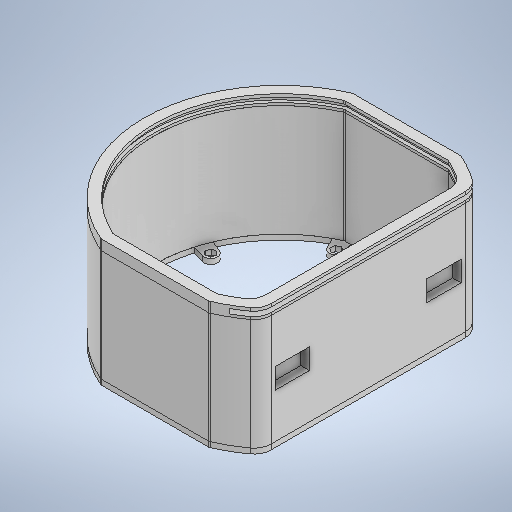
# Autodesk Inventor part: carcasa4.0
Saved by Autodesk Inventor 2025.3 (Build 293356030, 356C)
## iProperties
Created: 2025-08-27
Part Number: carcasa4.0
Material: Generic
Document SubType Name: Modeling
Designer: cdavi
Density: 1 g/cm^3
Appearance: Default
Author: cdavi
Autodesk Inventor part; units mm, degrees
ref_plane "YZ Plane" through (0, 0, 0) normal (1, 0, 0) x (0, 1, 0)
ref_plane "XZ Plane" through (0, 0, 0) normal (0, 1, 0) x (-1, 0, 0)
ref_plane "XY Plane" through (0, 0, 0) normal (0, 0, 1) x (1, 0, 0)
sketch "Sketch1" plane through (0, 0, 0) normal (0, 1, 0) x (-1, 0, 0)
  line L0 (29.8957, 67.5) -> (-29.8957, 67.5)
  line L1 (0, 0) -> (-51, 0) construction
  line L2 (31.1729, 73.5) -> (-31.1729, 73.5)
  line L3 (29.8957, -67.5) -> (-30.3274, -67.5)
  line L4 (31.1729, -73.5) -> (-31.1729, -73.5)
  line L5 (0, 0) -> (0, 73.5) construction
  line L6 (-45, 53.5817) -> (-45, -53.5817)
  line L7 (-51, 56.7362) -> (-51, -56.7362)
  arc A0 (-40.4687, -61.9539) -> (-30.3274, -67.5) centre (0, 0) ccw
  arc A1 (-46.8571, -64.8414) -> (-31.9722, -73.3333) centre (0, 0) ccw
  arc A2 (31.9722, -73.3333) -> (31.9722, 73.3333) centre (0, 0) ccw
  arc A3 (-31.9722, 73.3333) -> (-46.8571, 64.8414) centre (0, 0) ccw
  arc A4 (30.7261, -67.3194) -> (30.7261, 67.3194) centre (0, 0) ccw
  arc A5 (-30.7261, 67.3194) -> (-40.4688, 61.9539) centre (0, 0) ccw
  arc A6 (-31.9722, -73.3333) -> (-31.1729, -73.5) centre (-31.1729, -71.5) ccw
  arc A7 (31.1729, -73.5) -> (31.9722, -73.3333) centre (31.1729, -71.5) ccw
  arc A8 (29.8957, -67.5) -> (30.7261, -67.3194) centre (29.8957, -65.5) ccw
  arc A9 (30.7261, 67.3194) -> (29.8957, 67.5) centre (29.8957, 65.5) ccw
  arc A10 (31.9722, 73.3333) -> (31.1729, 73.5) centre (31.1729, 71.5) ccw
  arc A11 (-29.8957, 67.5) -> (-30.7261, 67.3194) centre (-29.8957, 65.5) ccw
  arc A12 (-31.1729, 73.5) -> (-31.9722, 73.3333) centre (-31.1729, 71.5) ccw
  arc A13 (-40.4688, 61.9539) -> (-45, 53.5817) centre (-35, 53.5817) ccw
  arc A14 (-46.8571, 64.8414) -> (-51, 56.7362) centre (-41, 56.7362) ccw
  arc A15 (-51, -56.7362) -> (-46.8571, -64.8414) centre (-41, -56.7362) ccw
  arc A16 (-45, -53.5817) -> (-40.4687, -61.9539) centre (-35, -53.5817) ccw
  point P0 (-31.5872, 73.5)
  point P1 (30.3274, -67.5)
  point P2 (31.5872, -73.5)
  point P3 (-31.5872, -73.5)
  point P4 (-51, -61.636)
  point P5 (-45, 58.7452)
  point P6 (-45, -58.7452)
  point P7 (-51, 61.636)
  point P8 (31.5872, 73.5)
  point P9 (30.3274, 67.5)
  point P10 (-30.3274, 67.5)
  dimension "d2" = 67.5
  dimension "d4" = 6
  dimension "d6" = 45
  dimension "d7" = 6
  dimension "d8" = 2
  dimension "d9" = 10
  dimension "d10" = 74
  dimension "d11" = 80
  dimension "d12" = 74
  dimension "d13" = 80
  constraints: 45 point on circle, 22 tangent, 17 centre point, 16 end point, 11 point on line, 9 equal radius, 4 symmetric about line, 3 vertical, 2 coincident, 2 horizontal, 2 midpoint, 1 parallel
  measures "d2" distance between parallel lines of L1 L0
  measures "d4" distance between parallel lines of L0 L2
  measures "d6" distance between parallel lines of L6 L5
  measures "d7" distance between parallel lines of L7 L6
  measures "d8" radius of A6
  measures "d9" radius of A13
  measures "d10" radius of A4
  measures "d11" radius of A2
  measures "d12" radius of A0
  measures "d13" radius of A1
extrude "Extrusion1" add sketch "Sketch1" along normal blind 65
sketch "Sketch2" plane through (51, 0, 56.7362) normal (1, 0, 0) x (0, 0, -1)
  line L0 (56.7362, 0) -> (56.7362, 65) construction
  line L1 (110.3179, 65) -> (3.1545, 65) projected
  line L2 (2.4029, 38) -> (22.4029, 38)
  line L3 (22.4029, 38) -> (22.4029, 26)
  line L4 (22.4029, 26) -> (2.4029, 26)
  line L5 (2.4029, 26) -> (2.4029, 38)
  line L6 (0, 0) -> (113.4725, 0) projected
  line L7 (-16.5971, 0) -> (-16.5971, 65) projected
  line L8 (111.0696, 38) -> (91.0696, 38)
  line L9 (91.0696, 38) -> (91.0696, 26)
  line L10 (91.0696, 26) -> (111.0696, 26)
  line L11 (111.0696, 26) -> (111.0696, 38)
  dimension "d16" = 26
  dimension "d17" = 19
  dimension "d18" = 12
  dimension "d19" = 20
  constraints: 18 end point, 4 symmetric about line, 2 parallel, 1 horizontal, 1 midpoint, 1 perpendicular
  measures "d16" distance between parallel lines of L6 L4
  measures "d17" distance between parallel lines of L5 L7
  measures "d18" distance of L2.end L3.end
  measures "d19" distance of L2.start L2.end
extrude "Extrusion2" cut sketch "Sketch2" against normal blind 5
sketch "Sketch3" plane through (51, 0, 56.7362) normal (1, 0, 0) x (0, 0, -1)
  line L0 (3.568, 49.2223) -> (17.7975, 43.9952) construction
  line L1 (2.8909, 47.379) -> (17.1204, 42.1519)
  line L2 (18.4746, 45.8385) -> (4.2452, 51.0656)
  arc A0 (4.2452, 51.0656) -> (2.8909, 47.379) centre (3.568, 49.2223) ccw
  arc A1 (17.1204, 42.1519) -> (18.4746, 45.8385) centre (17.7975, 43.9952) ccw
  arc A2 (44.4296, 11.624) -> (34.6921, 2.9774) centre (43.8866, 2.4292) ccw construction
  arc A3 (44.531, 13.3402) -> (32.9759, 3.0797) centre (43.8866, 2.4292) ccw
  arc A4 (44.3283, 9.9077) -> (36.4083, 2.8751) centre (43.8866, 2.4292) ccw
  arc A5 (44.3283, 9.9077) -> (44.531, 13.3402) centre (44.4296, 11.624) ccw
  arc A6 (32.9759, 3.0797) -> (36.4083, 2.8751) centre (34.6921, 2.9774) ccw
  line L3 (56.7362, 0) -> (56.7362, 65) construction
  line L4 (110.5816, 47.379) -> (96.3521, 42.1519)
  line L5 (94.9978, 45.8385) -> (109.2273, 51.0656)
  arc A7 (110.5816, 47.379) -> (109.2273, 51.0656) centre (109.9044, 49.2223) ccw
  arc A8 (94.9978, 45.8385) -> (96.3521, 42.1519) centre (95.675, 43.9952) ccw
  point P0 (10.6828, 46.6088)
  constraints: 18 point on circle, 12 end point, 9 centre point, 8 tangent, 6 symmetric about line, 1 midpoint, 1 parallel, 2 other
extrude "Extrusion3" [suppressed]
extrude "Extrusion4" add sketch "Sketch1" along normal blind 3 from surface at 65 separate body contours A9 A4 A8 L3 A0 A16 L6 A13 A5 A11 L0 | A10 A2 A7 L4 A6 A1 A15 L7 A14 A3 A12 L2
sketch "Sketch5" plane through (-31.1729, 68, 73.5) normal (0, 1, 0) x (1, 0, 0)
  circle A0 centre (31.1729, 73.5) radius 8.5
  circle A1 centre (1.1729, 73.5) radius 2.5
  line L0 (39.2969, 71) -> (48.1729, 71)
  line L1 (48.1729, 71) -> (48.1729, 76)
  line L2 (48.1729, 76) -> (39.2969, 76)
  line L3 (48.1729, 73.5) -> (82.1729, 73.5)
  line L4 (82.1729, 16.7638) -> (82.1729, 130.2362) projected
  line L5 (1.1729, 73.5) -> (-48.8271, 73.5)
  arc A2 (-0.7993, 146.8333) -> (-0.7993, 0.1667) centre (31.1729, 73.5) ccw projected
  dimension "d26" = 17
  dimension "d27" = 5
  dimension "d31" = 5
  dimension "d32" = 17
  dimension "d47" = 30
  dimension "d204" = 34
  dimension "d205" = 50
  dimension "d206" = 51
  constraints: 10 end point, 3 point on circle, 2 centre point, 2 horizontal alignment, 2 midpoint, 2 perpendicular, 1 coincident, 1 horizontal, 1 point on line
  measures "d26" diameter of A0
  measures "d27" diameter of A1
  measures "d31" distance between parallel lines of L2 L0
  measures "d32" distance from line of A0.centre L1
  measures "d47" distance of A0.centre L5.start
  measures "d204" distance of L3.start L3.end
  measures "d205" distance of L5.start L5.end
  measures "d206" distance from line of L4 point (31.173, 73.5)
extrude "Extrusion5" cut sketch "Sketch5" against normal through all bodies 2
sketch "Sketch6" plane through (0, 0, 0) normal (0, 1, 0) x (-1, 0, 0)
  circle A0 centre (0, 0) radius 67 construction
  arc A1 (-30.7261, 67.3194) -> (-40.4688, 61.9539) centre (0, 0) ccw projected
  arc A2 (-40.4688, 61.9539) -> (-45, 53.5817) centre (-35, 53.5817) ccw projected
  line L0 (-45, -53.5817) -> (-45, 53.5817) projected
  arc A3 (-45, -53.5817) -> (-40.4687, -61.9539) centre (-35, -53.5817) ccw projected
  arc A4 (-40.4687, -61.9539) -> (-30.3274, -67.5) centre (0, 0) ccw projected
  line L1 (29.8957, -67.5) -> (-30.3274, -67.5) construction
  arc A5 (30.7261, -67.3194) -> (30.7261, 67.3194) centre (0, 0) ccw projected
  line L2 (-29.8957, 67.5) -> (29.8957, 67.5) construction
  line L3 (31.1729, 73.5) -> (-31.1729, 73.5) projected
  arc A6 (-31.9722, 73.3333) -> (-46.8571, 64.8414) centre (0, 0) ccw projected
  arc A7 (-46.8571, 64.8414) -> (-51, 56.7362) centre (-41, 56.7362) ccw projected
  line L4 (-51, 56.7362) -> (-51, -56.7362) projected
  arc A8 (-51, -56.7362) -> (-46.8571, -64.8414) centre (-41, -56.7362) ccw projected
  arc A9 (-46.8571, -64.8414) -> (-31.9722, -73.3333) centre (0, 0) ccw projected
  line L5 (-31.1729, -73.5) -> (31.1729, -73.5) projected
  arc A10 (31.9722, -73.3333) -> (31.9722, 73.3333) centre (0, 0) ccw projected
  arc A11 (-29.4268, 61.303) -> (-37.1875, 56.9306) centre (0, 0) ccw construction
  arc A12 (-37.1875, 56.9306) -> (-39, 53.5817) centre (-35, 53.5817) ccw construction
  line L6 (-39, 53.5817) -> (-39, -53.5817) construction
  arc A13 (-39, -53.5817) -> (-37.1875, -56.9306) centre (-35, -53.5817) ccw construction
  arc A14 (-37.1875, -56.9306) -> (-29.4268, -61.303) centre (0, 0) ccw construction
  line L7 (-28.5613, -61.5) -> (28.5613, -61.5) construction
  line L8 (-28.5613, 61.5) -> (28.5613, 61.5) construction
  arc A15 (29.4268, -61.303) -> (29.4268, 61.303) centre (0, 0) ccw construction
  arc A16 (-8.124, -2.5) -> (-8.124, 2.5) centre (0, 0) ccw projected
  line L9 (0, 0) -> (63.1919, 22.2662) construction
  line L10 (0, 0) -> (80, 0) construction
  circle A17 centre (63.1919, 22.2662) radius 2.85 construction
  line L11 (0, 0) -> (0, -67) construction
  circle A18 centre (28.3154, 60.7226) radius 2.85 construction
  line L12 (28.3154, 60.7226) -> (0, 0) construction
  circle A19 centre (-41.5, 20) radius 2.85 construction
  circle A20 centre (-28.3154, 60.7226) radius 2.85 construction
  line L13 (-28.3154, 60.7226) -> (0, 0) construction
  arc A21 (-28.5613, 61.5) -> (-29.4268, 61.303) centre (-28.5613, 59.5) ccw construction
  arc A22 (-29.4268, -61.303) -> (-28.5613, -61.5) centre (-28.5613, -59.5) ccw construction
  arc A23 (28.5613, -61.5) -> (29.4268, -61.303) centre (28.5613, -59.5) ccw construction
  arc A24 (29.4268, 61.303) -> (28.5613, 61.5) centre (28.5613, 59.5) ccw construction
  arc A25 (-31.9722, -73.3333) -> (-31.1729, -73.5) centre (-31.1729, -71.5) ccw projected
  arc A26 (31.1729, -73.5) -> (31.9722, -73.3333) centre (31.1729, -71.5) ccw projected
  arc A27 (31.9722, 73.3333) -> (31.1729, 73.5) centre (31.1729, 71.5) ccw projected
  arc A28 (-31.1729, 73.5) -> (-31.9722, 73.3333) centre (-31.1729, 71.5) ccw projected
  circle A29 centre (63.1919, -22.2662) radius 2.85 construction
  circle A30 centre (28.3154, -60.7226) radius 2.85 construction
  circle A31 centre (-41.5, -20) radius 2.85 construction
  circle A32 centre (-28.3154, -60.7226) radius 2.85 construction
  line L14 (30.7261, 60.6622) -> (30.7261, 67.3194)
  line L15 (-30.7261, 60.6622) -> (-30.7261, 67.3194)
  line L16 (30.7261, 67.3194) -> (-30.7261, 67.3194)
  line L17 (30.7261, -60.6622) -> (30.7261, -67.3194)
  line L18 (-30.7261, -60.6622) -> (-30.7261, -67.3194)
  line L19 (30.7261, -67.3194) -> (-30.7261, -67.3194)
  circle A33 centre (63.1919, 22.2662) radius 4
  circle A34 centre (28.3154, 60.7226) radius 4
  line L20 (60.3905, 22.7899) -> (62.2448, 24.9542)
  line L21 (62.2448, 24.9542) -> (65.0462, 24.4304)
  line L22 (65.0462, 24.4304) -> (65.9934, 21.7424)
  line L23 (65.9934, 21.7424) -> (64.1391, 19.5782)
  line L24 (64.1391, 19.5782) -> (61.3376, 20.1019)
  line L25 (61.3376, 20.1019) -> (60.3905, 22.7899)
  line L26 (25.9808, 59.0879) -> (25.7324, 61.9271)
  line L27 (25.7324, 61.9271) -> (28.067, 63.5618)
  line L28 (28.067, 63.5618) -> (30.65, 62.3573)
  line L29 (30.65, 62.3573) -> (30.8984, 59.5182)
  line L30 (30.8984, 59.5182) -> (28.5638, 57.8835)
  line L31 (28.5638, 57.8835) -> (25.9808, 59.0879)
  circle A35 centre (-41.5, 20) radius 4
  line L32 (-43.9682, 18.575) -> (-43.9682, 21.425)
  line L33 (-43.9682, 21.425) -> (-41.5, 22.85)
  line L34 (-41.5, 22.85) -> (-39.0318, 21.425)
  line L35 (-39.0318, 21.425) -> (-39.0318, 18.575)
  line L36 (-39.0318, 18.575) -> (-41.5, 17.15)
  line L37 (-41.5, 17.15) -> (-43.9682, 18.575)
  line L38 (-41.5, 24) -> (-45, 24)
  line L39 (-41.5, 16) -> (-45, 16)
  circle A36 centre (-28.3154, 60.7226) radius 4
  line L40 (-28.5638, 57.8835) -> (-30.8984, 59.5182)
  line L41 (-30.8984, 59.5182) -> (-30.65, 62.3573)
  line L42 (-30.65, 62.3573) -> (-28.067, 63.5618)
  line L43 (-28.067, 63.5618) -> (-25.7324, 61.9271)
  line L44 (-25.7324, 61.9271) -> (-25.9808, 59.0879)
  line L45 (-25.9808, 59.0879) -> (-28.5638, 57.8835)
  line L46 (-31.8886, 58.9247) -> (-35.0362, 65.1802)
  circle A37 centre (63.1919, -22.2662) radius 4
  circle A38 centre (28.3154, -60.7226) radius 4
  circle A39 centre (-41.5, -20) radius 4
  line L47 (-41.5, -24) -> (-45, -24)
  line L48 (-41.5, -16) -> (-45, -16)
  circle A40 centre (-28.3154, -60.7226) radius 4
  line L49 (-31.8886, -58.9247) -> (-35.0362, -65.1802)
  line L50 (60.3905, -22.7899) -> (62.2448, -24.9542)
  line L51 (62.2448, -24.9542) -> (65.0462, -24.4304)
  line L52 (65.0462, -24.4304) -> (65.9934, -21.7424)
  line L53 (65.9934, -21.7424) -> (64.1391, -19.5782)
  line L54 (64.1391, -19.5782) -> (61.3376, -20.1019)
  line L55 (61.3376, -20.1019) -> (60.3905, -22.7899)
  line L56 (25.9808, -59.0879) -> (25.7324, -61.9271)
  line L57 (25.7324, -61.9271) -> (28.067, -63.5618)
  line L58 (28.067, -63.5618) -> (30.65, -62.3573)
  line L59 (30.65, -62.3573) -> (30.8984, -59.5182)
  line L60 (30.8984, -59.5182) -> (28.5638, -57.8835)
  line L61 (28.5638, -57.8835) -> (25.9808, -59.0879)
  line L62 (-28.5638, -57.8835) -> (-30.8984, -59.5182)
  line L63 (-30.8984, -59.5182) -> (-30.65, -62.3573)
  line L64 (-30.65, -62.3573) -> (-28.067, -63.5618)
  line L65 (-28.067, -63.5618) -> (-25.7324, -61.9271)
  line L66 (-25.7324, -61.9271) -> (-25.9808, -59.0879)
  line L67 (-25.9808, -59.0879) -> (-28.5638, -57.8835)
  line L68 (-43.9682, -18.575) -> (-43.9682, -21.425)
  line L69 (-43.9682, -21.425) -> (-41.5, -22.85)
  line L70 (-41.5, -22.85) -> (-39.0318, -21.425)
  line L71 (-39.0318, -21.425) -> (-39.0318, -18.575)
  line L72 (-39.0318, -18.575) -> (-41.5, -17.15)
  line L73 (-41.5, -17.15) -> (-43.9682, -18.575)
  line L74 (61.7506, 25.9975) -> (68.283, 28.5208)
  line L75 (64.408, 18.4555) -> (71.0794, 20.5846)
  line L76 (31.8886, 58.9247) -> (35.0362, 65.1802)
  line L77 (61.7506, -25.9975) -> (68.283, -28.5208)
  line L78 (64.408, -18.4555) -> (71.0794, -20.5846)
  line L79 (31.8886, -58.9247) -> (35.0362, -65.1802)
  line L80 (-24.6413, 62.3041) -> (-27.4101, 68.7364)
  line L81 (24.6413, 62.3041) -> (27.4101, 68.7364)
  line L82 (-24.6413, -62.3041) -> (-27.4101, -68.7364)
  line L83 (24.6413, -62.3041) -> (27.4101, -68.7364)
  line L84 (-29.8957, 67.5) -> (-51, 67.5)
  line L85 (-51, 67.5) -> (-51, 56.7362)
  line L86 (-42.9389, 67.5) -> (-29.8957, 67.5)
  point P0 (-29.0129, -61.5)
  point P1 (30.7261, -60.6622)
  point P2 (-30.7261, -60.6622)
  point P3 (28.3154, 60.7226)
  point P4 (28.3154, 60.7226)
  point P5 (-30.7261, -67.3194)
  point P6 (-35.0362, -65.1802)
  point P7 (71.0794, -20.5846)
  point P8 (68.283, -28.5208)
  point P9 (35.0362, -65.1802)
  point P10 (-27.1107, 64.5369)
  point P11 (-27.1107, -64.5369)
  point P12 (27.1107, -64.5369)
  point P13 (27.1107, 64.5369)
  point P14 (-45, 21.9365)
  point P15 (-45, 18.0635)
  point P16 (-32.0117, 62.2515)
  point P17 (32.0117, -62.2515)
  point P18 (66.8707, -20.6956)
  point P19 (65.0736, -25.796)
  point P20 (-32.0117, -62.2515)
  point P21 (-45, -21.9365)
  point P22 (-45, -18.0635)
  point P23 (65.0736, 25.796)
  point P24 (66.8707, 20.6956)
  point P25 (32.0117, 62.2515)
  point P26 (25.828, -65.0609)
  point P27 (-25.828, -65.0609)
  point P28 (30.7261, -63.9146)
  point P29 (-26.8002, -67.3194)
  point P30 (26.8002, -67.3194)
  point P31 (26.8002, 67.3194)
  point P32 (-26.8002, 67.3194)
  point P33 (30.7261, 63.9146)
  point P34 (-30.7261, -63.9146)
  point P35 (-30.7261, 63.9146)
  dimension "d33" = 134
  dimension "d39" = 5.7
  dimension "d34" = 6
  dimension "d35" = 6
  dimension "d36" = 6
  dimension "d37" = 19.41
  dimension "d38" = 25
  dimension "d40" = 20
  dimension "d41" = 3.5
  dimension "d42" = 25
  dimension "d44" = 2
  dimension "d61" = 8
  dimension "d62" = 8
  dimension "d63" = 8
  dimension "d64" = 8
  dimension "d171" = 90
  dimension "d172" = 10.7638
  constraints: 162 end point, 52 symmetric about line, 38 point on circle, 20 centre point, 16 tangent, 10 coincident, 6 perpendicular, 4 point on line, 3 equal radius, 2 parallel, 2 vertical, 1 collinear, 1 horizontal, 93 other
  measures "d34" radial gap between concentric circles of A1 A11
  measures "d35" distance between parallel lines of L2 L8
  measures "d36" radial gap between concentric circles of A5 A15
  measures "d37" angle of L10 L9
  measures "d38" angle of L11 L12
  measures "d40" distance from line of point (-41.5, 20) L10
  measures "d41" distance from line of L0 point (-41.5, 20)
  measures "d42" angle of L11 L13
  measures "d44" radius of A21
  measures "d61" diameter of A33
  measures "d62" diameter of A34
  measures "d63" diameter of A35
  measures "d64" diameter of A36
  measures "d171" angle of L85 L84
  measures "d172" distance of L84.end L4.start
extrude "Extrusion6" add sketch "Sketch6" against normal blind 3 separate body contours L15 A36 L46 A1 | L16 L80 A36 L15 | A36 | L16 L14 A34 L81 | A5 L76 A34 L14 | A34 | L38 A35 L0 | A35 L0 | L0 A35 | A5 L75 A33 L74 | A35 L39 L0 | A33 | A5 L77 A37 L78 | L48 A39 L0 | A37 | A39 L0 | L0 A39 | A5 L17 A38 L79 | A39 L47 L0 | L19 L83 A38 L17 | A38 | L19 L18 A40 L82 | A4 L49 A40 L18 | A40 | A27 A10 A26 L5 A25 A9 A8 L4 A7 A6 A28 L3
sketch "Sketch14" plane through (0, 65, 0) normal (0, 1, 0) x (1, 0, 0)
  arc A0 (-31.9722, 73.3333) -> (-31.9722, -73.3333) centre (0, 0) ccw projected
  arc A1 (-31.9722, -73.3333) -> (-31.1729, -73.5) centre (-31.1729, -71.5) ccw projected
  line L0 (-31.1729, -73.5) -> (31.1729, -73.5) projected
  arc A2 (31.1729, -73.5) -> (31.9722, -73.3333) centre (31.1729, -71.5) ccw projected
  arc A3 (31.9722, -73.3333) -> (46.8571, -64.8414) centre (0, 0) ccw projected
  arc A4 (46.8571, -64.8414) -> (51, -56.7362) centre (41, -56.7362) ccw projected
  line L1 (51, -56.7362) -> (51, 56.7362) projected
  arc A5 (51, 56.7362) -> (46.8571, 64.8414) centre (41, 56.7362) ccw projected
  arc A6 (46.8571, 64.8414) -> (31.9722, 73.3333) centre (0, 0) ccw projected
  arc A7 (31.9722, 73.3333) -> (31.1729, 73.5) centre (31.1729, 71.5) ccw projected
  line L2 (31.1729, 73.5) -> (-31.1729, 73.5) projected
  arc A8 (-31.1729, 73.5) -> (-31.9722, 73.3333) centre (-31.1729, 71.5) ccw projected
  line L3 (-29.8957, 67.5) -> (30.3274, 67.5) projected
  arc A9 (40.4687, 61.9539) -> (30.3274, 67.5) centre (0, 0) ccw projected
  arc A10 (45, 53.5817) -> (40.4687, 61.9539) centre (35, 53.5817) ccw projected
  line L4 (45, 53.5817) -> (45, -53.5817) projected
  arc A11 (40.4688, -61.9539) -> (45, -53.5817) centre (35, -53.5817) ccw projected
  arc A12 (30.7261, -67.3194) -> (40.4688, -61.9539) centre (0, 0) ccw projected
  arc A13 (29.8957, -67.5) -> (30.7261, -67.3194) centre (29.8957, -65.5) ccw projected
  line L5 (29.8957, -67.5) -> (-29.8957, -67.5) projected
  arc A14 (-30.7261, -67.3194) -> (-29.8957, -67.5) centre (-29.8957, -65.5) ccw projected
  arc A15 (-30.7261, 67.3194) -> (-30.7261, -67.3194) centre (0, 0) ccw projected
  arc A16 (-29.8957, 67.5) -> (-30.7261, 67.3194) centre (-29.8957, 65.5) ccw projected
extrude "Extrusion11" add sketch "Sketch14" along normal blind 6 separate body
sketch "Sketch15" plane through (51, 65, 56.7362) normal (1, 0, 0) x (0, 0, -1)
  line L0 (56.7362, 6) -> (56.7362, 0)
  line L1 (56.7362, 6) -> (0, 6)
  line L2 (0, 6) -> (-12.763, 6)
  line L3 (-12.763, 6) -> (-12.763, 0)
  line L4 (-12.763, 0) -> (0, 0)
  line L5 (0, 0) -> (56.7362, 0)
  line L6 (3.1545, 0) -> (56.7362, 0)
  line L7 (56.7362, 6) -> (0, 6)
  line L8 (56.7362, 6) -> (56.7362, 4.5)
  line L9 (56.7362, 4.5) -> (0, 4.246)
  line L10 (0, 0) -> (0, 6) projected
  line L11 (56.7362, 0) -> (56.7362, 1.5)
  line L12 (56.7362, 1.5) -> (0, 1.5)
  arc A0 (56.7362, 4.5) -> (56.7362, 4.5) centre (56.0237, 163.6579) ccw
  line L13 (0, 4.246) -> (-12.763, 4.246)
  line L14 (0, 1.5) -> (-12.763, 1.5)
  line L15 (56.7362, 6) -> (113.4725, 6)
  line L16 (113.4725, 6) -> (126.2355, 6)
  line L17 (126.2355, 6) -> (126.2355, 0)
  line L18 (126.2355, 0) -> (113.4725, 0)
  line L19 (113.4725, 0) -> (56.7362, 0)
  line L20 (110.3179, 0) -> (56.7362, 0)
  line L21 (56.7362, 6) -> (113.4725, 6)
  line L22 (56.7362, 4.5) -> (113.4725, 4.246)
  line L23 (113.4725, 0) -> (113.4725, 6)
  line L24 (56.7362, 1.5) -> (113.4725, 1.5)
  arc A1 (56.7362, 4.5) -> (56.7362, 4.5) centre (57.4488, 163.6579) ccw
  line L25 (113.4725, 4.246) -> (126.2355, 4.246)
  line L26 (113.4725, 1.5) -> (126.2355, 1.5)
  point P0 (56.7362, -65)
  dimension "d173" = 12.763
  dimension "d176" = 1.5
  dimension "d177" = 1.5
  dimension "d202" = 2.746
  constraints: 52 end point, 15 point on line, 11 symmetric about line, 6 perpendicular, 4 point on circle, 2 centre point, 1 collinear, 1 tangent, 1 other
  measures "d173" distance of L1.end L2.end
  measures "d176" distance of L0.start L8.end
  measures "d177" distance of L0.end L11.end
  measures "d202" distance between parallel lines of L14 L13
extrude "Extrusion12" cut sketch "Sketch15" against normal blind 82.146 contours L22 L23 L24 L0 | L0 L12 L10 L9 | L10 L14 L3 L13 | L25 L17 L26 L23 bodies 4
ref_plane "Work Plane1" through (0, 66.5, 0) normal (0, -1, 0) x (1, 0, 0)
sketch "Sketch18" plane through (0, 66.5, 0) normal (0, -1, 0) x (1, 0, 0)
  arc A0 (-29.8957, 67.6923) -> (-29.8957, -67.6923) centre (0, 0) ccw
  arc A1 (-29.8957, 69.8731) -> (-29.8957, -69.8731) centre (0, 0) ccw
  line L0 (30.3274, -67.5) -> (-29.8957, -67.5) projected
  line L1 (-29.8957, -67.5) -> (-29.8957, -69.8731)
  line L2 (-29.8957, 67.5) -> (29.8957, 67.5) projected
  line L3 (-29.8957, 67.5) -> (-29.8957, 69.8731)
  point P0 (-30.7261, -67.3194)
  point P1 (-30.7261, 67.3194)
  point P2 (-29.896, -69.4992)
  dimension "d199" = 152
  constraints: 5 end point, 4 point on circle, 2 centre point, 2 coincident, 2 point on line, 1 perpendicular, 1 vertical
  measures "d199" diameter of A1
extrude "Extrusion14" cut sketch "Sketch18" against normal blind 2.746 bodies 4
body "Solid1"
body "Solid2"
body "Solid3"
body "Solid4"
